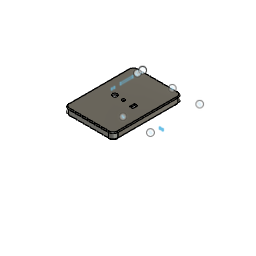
enclosure_part2 (Autodesk Fusion 360 design; units mm, degrees)
Autodesk Fusion 360 part; units mm, degrees
note: some values were not read from the file. Chosen so that the rebuilt part matches the saved one: where a step ends.
sketch "Sketch1" plane through (51.7, -43.8, 7) normal (0, 0, 1) x (0, -1, 0)
  line L0 (-40.66, -52.3) -> (-41.86, -52.3)
  line L1 (-41.86, -52.3) -> (-41.86, -51.1)
  line L2 (-41.86, -51.1) -> (-40.66, -51.1)
  line L3 (-40.66, -51.1) -> (-40.66, -52.3)
  line L4 (-39.32, -52.3) -> (-39.32, -51.1)
  line L5 (-39.32, -51.1) -> (-38.12, -51.1)
  line L6 (-38.12, -51.1) -> (-38.12, -52.3)
  line L7 (-38.12, -52.3) -> (-39.32, -52.3)
  line L8 (-43.2, -51.1) -> (-43.2, -52.3)
  line L9 (-43.2, -52.3) -> (-44.4, -52.3)
  line L10 (-44.4, -52.3) -> (-44.4, -51.1)
  line L11 (-44.4, -51.1) -> (-43.2, -51.1)
  line L12 (-35.58, -51.1) -> (-35.58, -52.3)
  line L13 (-35.58, -52.3) -> (-36.78, -52.3)
  line L14 (-36.78, -52.3) -> (-36.78, -51.1)
  line L15 (-36.78, -51.1) -> (-35.58, -51.1)
  line L16 (-80, -3) -> (-80, -52)
  line L17 (-77, -55) -> (-3, -55)
  arc A0 (-80, -52) -> (-77, -55) centre (-77, -52) ccw
  circle A1 centre (-77, -52) radius 1.1
  arc A2 (-77, 0) -> (-80, -3) centre (-77, -3) ccw
  line L18 (-3, 0) -> (-77, 0)
  arc A3 (-3, -55) -> (0, -52) centre (-3, -52) ccw
  circle A4 centre (-3, -52) radius 1.1
  line L19 (0, -52) -> (0, -3)
  arc A5 (0, -3) -> (-3, 0) centre (-3, -3) ccw
  circle A6 centre (-3, -3) radius 1.1
  circle A7 centre (-77, -3) radius 1.1
  line L20 (1, -52) -> (1, -3)
  arc A8 (1, -3) -> (-3, 1) centre (-3, -3) ccw
  line L21 (-3, 1) -> (-77, 1)
  arc A9 (-77, 1) -> (-81, -3) centre (-77, -3) ccw
  line L22 (-81, -3) -> (-81, -52)
  arc A10 (-81, -52) -> (-77, -56) centre (-77, -52) ccw
  line L23 (-77, -56) -> (-3, -56)
  arc A11 (-3, -56) -> (1, -52) centre (-3, -52) ccw
  line L24 (-3, 3) -> (-77, 3)
  arc A12 (-77, 3) -> (-83, -3) centre (-77, -3) ccw
  line L25 (-83, -3) -> (-83, -52)
  arc A13 (-83, -52) -> (-77, -58) centre (-77, -52) ccw
  line L26 (-77, -58) -> (-3, -58)
  arc A14 (-3, -58) -> (3, -52) centre (-3, -52) ccw
  line L27 (3, -52) -> (3, -3)
  arc A15 (3, -3) -> (-3, 3) centre (-3, -3) ccw
  circle A16 centre (-40.0821, -27.3917) radius 1.3
  circle A17 centre (-40.0821, -27.3917) radius 1.9
  circle A18 centre (-40.095, -38) radius 2.5
  circle A19 centre (-40.095, -38) radius 3
  line L28 (-37.5, -16.0948) -> (-42.5, -16.0948) construction
  line L29 (-42.5, -16.0948) -> (-42.5, -13.0948) construction
  line L30 (-42.5, -13.0948) -> (-37.5, -13.0948) construction
  line L31 (-37.5, -13.0948) -> (-37.5, -16.0948) construction
  line L32 (-5.0576, 1) -> (-4.9998, -3.0287)
  line L33 (-3, -5) -> (1, -5)
  line L34 (-40, 3) -> (-40, -58) construction
  line L35 (-83, -27.5) -> (3, -27.5) construction
  arc A20 (-4.9998, -3.0287) -> (-3, -5) centre (-3, -3) ccw
  line L36 (-74.9424, 1) -> (-75.0002, -3.0287)
  arc A21 (-77, -5) -> (-75.0002, -3.0287) centre (-77, -3) ccw
  line L37 (-77, -5) -> (-81, -5)
  line L38 (-5.0576, -56) -> (-4.9998, -51.9713)
  arc A22 (-3, -50) -> (-4.9998, -51.9713) centre (-3, -52) ccw
  line L39 (-3, -50) -> (1, -50)
  line L40 (-74.9424, -56) -> (-75.0002, -51.9713)
  arc A23 (-75.0002, -51.9713) -> (-77, -50) centre (-77, -52) ccw
  line L41 (-77, -50) -> (-81, -50)
  circle A24 centre (-3, -3) radius 1.1
  circle A25 centre (-77, -3) radius 1.1
  circle A26 centre (-3, -52) radius 1.1
  circle A27 centre (-77, -52) radius 1.1
  line L42 (-43, -16.5948) -> (-43, -12.5948)
  line L43 (-43, -12.5948) -> (-37, -12.5948)
  line L44 (-37, -12.5948) -> (-37, -16.5948)
  line L45 (-37, -16.5948) -> (-43, -16.5948)
  dimension "d1" = 1
  dimension "d4" = 3
  dimension "d8" = 4
  dimension "d9" = 3.8
  dimension "d10" = 6
  dimension "d11" = 5
  dimension "d12" = 3
  dimension "d19" = -0.5
  constraint concentric A5 A20
  constraint concentric A16 A17
  constraint concentric A18 A19
  constraint horizontal L28
  constraint vertical L29
  constraint horizontal L30
  constraint vertical L31
  constraint coincident L21 L32.start
  constraint tangent L32 A20
  constraint coincident L20 L33.end
  constraint perpendicular L20 L33
  constraint midpoint L24 L34.start
  constraint midpoint L26 L34.end
  constraint midpoint L25 L35.start
  constraint midpoint L27 L35.end
  constraint tangent L33 A20
  constraint symmetric L32.start L34 L36.start
  constraint symmetric L32.end L34 L36.end
  constraint symmetric L33.start L34 A21.start
  constraint symmetric L33.end L34 L37.end
  constraint symmetric L34 A20 A21
  constraint symmetric L32.start L35 L38.start
  constraint symmetric L32.end L35 L38.end
  constraint symmetric L33.start L35 A22.start
  constraint symmetric L33.end L35 L39.end
  constraint symmetric L35 A20 A22
  constraint symmetric L35 L36.start L40.start
  constraint symmetric L35 L36.end L40.end
  constraint symmetric L35 A21.start A23.end
  constraint symmetric L35 A21 A23
  constraint symmetric L35 L37.end L41.end
  constraint concentric A5 A24
  constraint symmetric L34 A24 A25
  constraint symmetric L35 A24 A26
  constraint symmetric L35 A25 A27
  measures "d8" diameter of A20
  measures "d9" diameter of A17
  measures "d10" diameter of A19
  measures "d11" distance of L28.start L28.end
  measures "d12" distance of L28.start L30.end
extrude "Extrude1" add sketch "Sketch1" against normal up to surface (4.7767 mm away) contours L24 A12 L25 A13 L26 A14 L27 A15 makes body 1
extrude "Extrude2" add sketch "Sketch1" along normal blind 2 contours L0 L1 L2 L3 | L4 L5 L6 L7 | L8 L9 L10 L11 | L12 L13 L14 L15 | L16 A2 L18 L36 A21 L37 | L16 A2 L18 L21 A9 L22 L36 L37 | L16 L17 L18 L19 L32 L33 A20 L36 A21 L37 L38 A22 L39 L40 A23 L41 | L16 L22 L37 L41 | L16 L17 A0 L40 A23 L41 | L16 L17 A0 L22 A10 L23 L40 L41 | L18 L21 L32 L36 | L18 L19 A5 L20 A8 L21 L32 L33 | L18 L19 A5 L32 L33 A20 | L17 L23 L38 L40 | L17 A3 L19 L38 A22 L39 | L17 A3 L19 L20 L23 A11 L38 L39 | L19 L20 L33 L39 | A1 A27 | A4 A26 | A6 A24 | A7 A25 | L24 A12 L25 A13 L26 A14 L27 A15 bodies 1
extrude "Extrude3" add sketch "Sketch1" against normal blind 7 separate body contours L16 A2 L18 L36 A21 L37 | L16 A2 L18 L21 A9 L22 L36 L37 | L16 L17 A0 L40 A23 L41 | L16 L17 A0 L22 A10 L23 L40 L41 | L18 L19 A5 L20 A8 L21 L32 L33 | L18 L19 A5 L32 L33 A20 | L17 A3 L19 L38 A22 L39 | L17 A3 L19 L20 L23 A11 L38 L39 makes body 2 at (-0.4095, -41.8945, 2.3333) makes body 3 at (48.5905, 32.1055, 2.3333) makes body 4 at (48.5905, -41.8945, 2.3333) makes body 5 at (-0.8261, 34.166, 2.3333)
fillet "Fillet1" radius 1 8 edges at (24.2, 39.2, 9) (-4.5426, 37.4426, 9) (-6.3, -3.8, 9) (-4.5426, -45.0426, 9) (24.2, -46.8, 9) (52.9426, -45.0426, 9) (54.7, -3.8, 9) (52.9426, 37.4426, 9) on bodies 1
sketch "sketch 1895" plane through (-3, 0, 0) normal (-1, 0, 0) x (0, -1, 0)
  line L0 (-20, 0) -> (-35, 0)
  line L1 (-20, 2) -> (-20, 0)
  line L2 (-35, 2) -> (-20, 2)
  line L3 (-35, 0) -> (-35, 2)
  line L4 (-9, 0) -> (-12.5, 0)
  line L5 (-9, 1.5) -> (-9, 0)
  line L6 (-12.5, 1.5) -> (-9, 1.5)
  line L7 (-12.5, 0) -> (-12.5, 1.5)
  arc A0 (-40.96, -0.3) -> (-39.18, 1.48) centre (-40.96, 1.48) ccw
  line L8 (-39.18, 1.48) -> (-39.18, 2.08)
  arc A1 (-39.18, 2.08) -> (-40.96, 3.86) centre (-40.96, 2.08) ccw
  line L9 (-40.96, 3.86) -> (-47.34, 3.86)
  arc A2 (-47.34, 3.86) -> (-49.12, 2.08) centre (-47.34, 2.08) ccw
  line L10 (-49.12, 2.08) -> (-49.12, 1.48)
  arc A3 (-49.12, 1.48) -> (-47.34, -0.3) centre (-47.34, 1.48) ccw
  line L11 (-47.34, -0.3) -> (-44.65, -0.3)
  line L12 (-44.6, -0.3) -> (-44.65, -0.3)
  line L13 (-44.6, -0.3) -> (-40.96, -0.3)
extrude "Extrude4" cut sketch "sketch 1895" along normal up to near side of body 1 bodies 1
sketch "sketch 1969" plane through (0, -3, 0) normal (0, -1, 0) x (1, 0, 0)
  circle A0 centre (23, -9.9563) radius 1
  circle A1 centre (57, -9.9563) radius 1
extrude "Extrude5" cut sketch "sketch 1969" against normal up to surface (6 mm away) bodies 1
sketch "sketch 1996" plane through (0, 58, 0) normal (0, 1, 0) x (-1, 0, 0)
  circle A0 centre (-57, -9.9563) radius 1
  circle A1 centre (-23, -9.9563) radius 1
extrude "Extrude6" cut sketch "sketch 1996" against normal up to surface (6 mm away) bodies 1
sketch "sketch 2023" plane through (0, -3, 0) normal (0, -1, 0) x (1, 0, 0)
  line L0 (72.3452, 0.0156) -> (68.6651, 0.0156)
  line L1 (72.3452, 1.4876) -> (72.3452, 0.0156)
  line L2 (68.6651, 1.4876) -> (72.3452, 1.4876)
  line L3 (68.6651, 0.0156) -> (68.6651, 1.4876)
extrude "Extrude7" cut sketch "sketch 2023" along normal up to near side of body 1 bodies 1
equation "d4 = margin + wall_thickness"
equation "d15 = wall_thickness"
equation "d17 = -boss_height"
equation "d19 = -margin / 2"
equation "d43 = fillet_radius"
equation "margin = 1 mm"
equation "wall_thickness = 2 mm"
equation "boss_height = 7 mm"
equation "fillet_radius = 1 mm"
